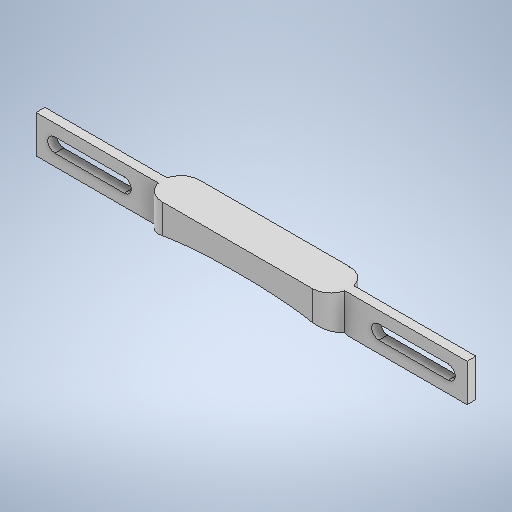
# Autodesk Inventor part: AllFretBars
Saved by Autodesk Inventor 2025.1 (Build 291241000, 241)
## iProperties
Created: 2025-11-05
Part Number: AllFretBars
Material: Generic
Document SubType Name: Modeling
Designer: Juxin
Density: 1 g/cm^3
Appearance: Default
Author: Juxin
Autodesk Inventor part; units mm, degrees
ref_plane "YZ Plane" through (0, 0, 0) normal (1, 0, 0) x (0, 1, 0)
ref_plane "XZ Plane" through (0, 0, 0) normal (0, 1, 0) x (-1, 0, 0)
ref_plane "XY Plane" through (0, 0, 0) normal (0, 0, 1) x (1, 0, 0)
sketch "Sketch1" plane through (0, 0, 0) normal (0, 1, 0) x (-1, 0, 0)
  line L0 (77.4625, -7.85) -> (77.4625, -4.85)
  line L1 (0, 0) -> (17.4625, 0) construction
  line L2 (77.4625, -6.35) -> (77.4625, -4.85)
  line L3 (77.4625, -4.85) -> (61.5875, -4.85)
  line L4 (61.5875, -7.85) -> (77.4625, -7.85)
  line L5 (61.5875, -4.85) -> (61.5875, 0)
  line L6 (61.5875, -7.85) -> (61.5875, -12.7)
  line L7 (61.5875, 0) -> (30, 0)
  line L8 (61.5875, -12.7) -> (30, -12.7)
  line L9 (-17.4625, -7.85) -> (-17.4625, -4.85)
  line L10 (-17.4625, -6.35) -> (-17.4625, -4.85)
  line L11 (-17.4625, -4.85) -> (-1.5875, -4.85)
  line L12 (-1.5875, -7.85) -> (-17.4625, -7.85)
  line L13 (-1.5875, -4.85) -> (-1.5875, 0)
  line L14 (-1.5875, -7.85) -> (-1.5875, -12.7)
  line L15 (-1.5875, 0) -> (30, 0)
  line L16 (-1.5875, -12.7) -> (30, -12.7)
  dimension "d23" = 1.5
  dimension "d24" = 15.875
  dimension "d25" = 3
  dimension "d27" = 63.175
  dimension "d117" = 12.7
  constraints: 34 end point, 2 horizontal, 2 midpoint, 2 perpendicular, 2 point on line
  measures "d23" distance of L0.end L2.start
  measures "d24" distance of L0.end L3.end
  measures "d25" distance of L3.end L4.start
  measures "d27" distance of L13.end L5.end
  measures "d117" distance of L6.end L5.end
extrude "Extrusion1" add sketch "Sketch1" along normal blind 12.7
sketch "Sketch3" plane through (1.5875, 0, -12.7) normal (0, 0, -1) x (-1, 0, 0)
  line L0 (0, 0) -> (63.175, 0) projected
  ellipse E0 centre (31.5875, 0) end of major axis (31.5875, 4.6466) minor radius 31.5875
  point P0 (1.5875, 0)
  constraints: 1 horizontal alignment, 1 midpoint, 2 other
extrude "Extrusion15" cut sketch "Sketch3" against normal blind 20.6375
fillet "Fillet2" radius 6.35 4 edges at (1.5875, 6.35, -12.7) (-61.5875, 6.35, -12.7) (-61.5875, 6.35, 0) (1.5875, 6.35, 0)
move faces "Move1" translate (25.4, 0, 0) faces at (17.4625, 4.2333, -5.85)
move faces "Move2" translate (-25.4, 0, 0) faces at (-77.4625, 4.2333, -6.85)
sketch "Sketch5" plane through (-61.5875, 0, -7.85) normal (0, 0, -1) x (-1, 0, 0)
  line L0 (-63.175, 0) -> (-63.175, 12.7) projected
  line L1 (-63.175, 6.35) -> (-74.605, 6.35)
  arc A0 (-74.605, 3.9688) -> (-74.605, 8.7312) centre (-74.605, 6.35) ccw
  line L2 (-104.45, 0) -> (-104.45, 12.7) projected
  line L3 (-104.45, 6.35) -> (-98.1, 6.35)
  arc A1 (-98.1, 8.7312) -> (-98.1, 3.9688) centre (-98.1, 6.35) ccw
  line L4 (-98.1, 3.9688) -> (-74.605, 3.9688)
  line L5 (-74.605, 8.7312) -> (-98.1, 8.7312)
  line L6 (-57.0047, 12.7) -> (-6.1703, 12.7) projected
  line L7 (-31.5875, 12.7) -> (-31.5875, 0)
  arc A2 (11.43, 8.7312) -> (11.43, 3.9688) centre (11.43, 6.35) ccw
  arc A3 (34.925, 3.9688) -> (34.925, 8.7312) centre (34.925, 6.35) ccw
  line L8 (34.925, 3.9688) -> (11.43, 3.9688)
  line L9 (11.43, 8.7312) -> (34.925, 8.7312)
  point P0 (-61.5875, 0)
  dimension "d126" = 11.43
  dimension "d127" = 4.7625
  dimension "d128" = 6.35
  dimension "d129" = 4.7625
  constraints: 14 end point, 8 point on circle, 6 symmetric about line, 4 centre point, 3 midpoint, 2 coincident, 2 horizontal, 2 tangent, 1 vertical, 2 other
  measures "d126" distance of L1.start L1.end
  measures "d127" diameter of A0
  measures "d128" distance of L3.start L3.end
  measures "d129" diameter of A1
extrude "Extrusion17" cut sketch "Sketch5" against normal blind 25.4
fillet "Fillet3" radius 3.175 2 edges at (1.5875, 0, -6.35) (-61.5875, 0, -6.35)
body "Solid1"
